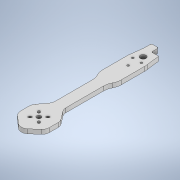
# Autodesk Inventor part: TokerCNC froggy arm
Saved by Autodesk Inventor 2020 (Build 240168000, 168)
## iProperties
Created: 2022-08-18
Part Number: TokerCNC froggy arm
Material: Generic
Document SubType Name: Modeling
Designer: Steven
Density: 1 g/cm^3
Appearance: Default
Author: Steven
Autodesk Inventor part; units mm, degrees
ref_plane "YZ Plane" through (0, 0, 0) normal (1, 0, 0) x (0, 1, 0)
ref_plane "XZ Plane" through (0, 0, 0) normal (0, 1, 0) x (-1, 0, 0)
ref_plane "XY Plane" through (0, 0, 0) normal (0, 0, 1) x (1, 0, 0)
sketch "Sketch1" plane through (0, 0, 0) normal (0, 1, 0) x (-1, 0, 0)
  line L0 (0, -158) -> (0, -165)
  arc A0 (1.5, -166.5) -> (0, -165) centre (0, -166.5) ccw
  line L1 (1.5, -166.5) -> (8.5, -166.5)
  arc A1 (8.5, -166.5) -> (10, -165) centre (8.5, -165) ccw
  line L2 (10, -165) -> (10, -156.5)
  line L3 (10, -156.5) -> (12.2297, -138.6622)
  arc A2 (12.2297, -138.6622) -> (12.5, -134.321) centre (-22.5, -134.321) ccw
  line L4 (12.5, -134.321) -> (12.5, -101.0909)
  arc A3 (12.5, -101.0909) -> (10.05, -91.4994) centre (-7.5, -101.0909) ccw
  arc A4 (7.6, -81.9079) -> (10.05, -91.4994) centre (27.6, -81.9079) ccw
  line L5 (7.6, -81.9079) -> (7.6, -29.8667)
  arc A5 (9.6, -23.8667) -> (7.6, -29.8667) centre (17.6, -29.8667) ccw
  line L6 (9.6, -23.8667) -> (18, -12.6667)
  arc A6 (18, -12.6667) -> (20, -6.6667) centre (10, -6.6667) ccw
  line L7 (20, -6.6667) -> (20, 5.4953)
  arc A7 (20, 5.4953) -> (16.6262, 12.9849) centre (10, 5.4953) ccw
  line L8 (16.6262, 12.9849) -> (6.6262, 21.8321)
  arc A8 (6.6262, 21.8321) -> (-6.6262, 21.8321) centre (0, 14.3426) ccw
  line L9 (-6.6262, 21.8321) -> (-16.6262, 12.9849)
  arc A9 (-16.6262, 12.9849) -> (-20, 5.4953) centre (-10, 5.4953) ccw
  line L10 (-20, 5.4953) -> (-20, -6.6667)
  arc A10 (-20, -6.6667) -> (-18, -12.6667) centre (-10, -6.6667) ccw
  line L11 (-18, -12.6667) -> (-9.6, -23.8667)
  arc A11 (-7.6, -29.8667) -> (-9.6, -23.8667) centre (-17.6, -29.8667) ccw
  line L12 (-7.6, -29.8667) -> (-7.6, -82.5915)
  arc A12 (-10.05, -92.183) -> (-7.6, -82.5915) centre (-27.6, -82.5915) ccw
  arc A13 (-10.05, -92.183) -> (-12.5, -101.7745) centre (7.5, -101.7745) ccw
  line L13 (-12.5, -101.7745) -> (-12.5, -134.321)
  arc A14 (-12.5, -134.321) -> (-12.2297, -138.6622) centre (22.5, -134.321) ccw
  line L14 (-12.2297, -138.6622) -> (-10, -156.5)
  line L15 (-10, -156.5) -> (-1.5, -156.5)
  arc A15 (0, -158) -> (-1.5, -156.5) centre (-1.5, -158) ccw
  arc A16 (-6.7529, 4.5608) -> (-4.5608, 6.7529) centre (-5.6569, 5.6569) ccw
  line L16 (-4.5608, 6.7529) -> (-5.6215, 7.8135)
  arc A17 (-5.6215, 7.8135) -> (-7.8135, 5.6215) centre (-6.7175, 6.7175) ccw
  line L17 (-7.8135, 5.6215) -> (-6.7529, 4.5608)
  line L18 (6.7529, -4.5608) -> (7.8135, -5.6215)
  arc A18 (5.6215, -7.8135) -> (7.8135, -5.6215) centre (6.7175, -6.7175) ccw
  line L19 (5.6215, -7.8135) -> (4.5608, -6.7529)
  arc A19 (6.7529, -4.5608) -> (4.5608, -6.7529) centre (5.6569, -5.6569) ccw
  line L20 (-7.8135, -5.6215) -> (-6.7529, -4.5608)
  arc A20 (-4.5608, -6.7529) -> (-6.7529, -4.5608) centre (-5.6569, -5.6569) ccw
  line L21 (-4.5608, -6.7529) -> (-5.6215, -7.8135)
  arc A21 (-7.8135, -5.6215) -> (-5.6215, -7.8135) centre (-6.7175, -6.7175) ccw
  line L22 (7.8135, 5.6215) -> (6.7529, 4.5608)
  arc A22 (4.5608, 6.7529) -> (6.7529, 4.5608) centre (5.6569, 5.6569) ccw
  line L23 (4.5608, 6.7529) -> (5.6215, 7.8135)
  arc A23 (7.8135, 5.6215) -> (5.6215, 7.8135) centre (6.7175, 6.7175) ccw
  circle A24 centre (0, 0) radius 3
  circle A25 centre (0, -124.0736) radius 1.5
  circle A26 centre (-6, -136.5) radius 1.5
  circle A27 centre (6, -136.5) radius 1.5
  circle A28 centre (0, -144.9332) radius 4
  point P0 (10, -165)
  point P1 (12.2297, -138.6622)
  point P2 (12.5, -101.0909)
  point P3 (10.05, -91.4994)
  point P4 (7.6, -81.9079)
  point P5 (7.6, -29.8667)
  point P6 (9.6, -23.8667)
  point P7 (20, -6.6667)
  point P8 (20, 5.4953)
  point P9 (16.6262, 12.9849)
  point P10 (6.6262, 21.8321)
  point P11 (-16.6262, 12.9849)
  point P12 (-20, 5.4953)
  point P13 (-9.6, -23.8667)
  point P14 (-10.05, -92.183)
  point P15 (-12.2297, -138.6622)
  point P16 (0, -158)
  point P17 (6.7529, -4.5608)
  point P18 (7.8135, -5.6215)
  point P19 (5.6215, -7.8135)
  point P20 (-7.8135, -5.6215)
  point P21 (-6.7529, -4.5608)
  point P22 (-4.5608, -6.7529)
  point P23 (-5.6215, -7.8135)
  point P24 (-5.6215, 7.8135)
  point P25 (-4.5608, 6.7529)
  constraints: 48 end point, 48 point on circle, 29 centre point
extrude "Extrusion1" add sketch "Sketch1" along normal blind 6
body "Solid1"
